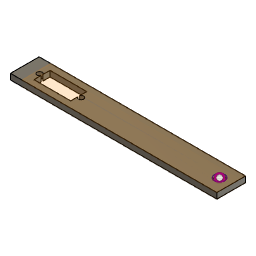
mechanical parts design (Autodesk Fusion 360 archive; units mm, degrees)
design "bar 1"
Autodesk Fusion 360 part; units mm, degrees
note: some values were not read from the file. Set by a fixed rule: which sketch regions a step uses.
sketch "Sketch1" plane through (0, 0, 0) normal (0, 1, 0) x (1, 0, 0)
  line L0 (0, 25) -> (170, 25)
  line L1 (170, 25) -> (170, 0)
  line L2 (170, 0) -> (0, 0)
  line L3 (0, 0) -> (0, 25)
  dimension "d1" = 170
  dimension "d2" = 25
  constraint horizontal L0
  constraint vertical L1
  constraint horizontal L2
  constraint vertical L3
  measures "d1" distance of L0.start L0.end
  measures "d2" distance of L0.end L1.end
extrude "Extrude1" add sketch "Sketch1" along normal blind 5
sketch "Sketch2" plane through (0, 5, 0) normal (0, 1, 0) x (-1, 0, 0)
  line L0 (0, 0) -> (-170, 0)
  line L1 (-170, 0) -> (-170, -25)
  line L2 (-170, -25) -> (0, -25)
  line L3 (0, -25) -> (0, 0)
  line L4 (0, -12.5) -> (-170, -12.5) construction
  line L5 (-5, -19.5) -> (-37, -19.5)
  line L6 (-37, -19.5) -> (-37, -5.5)
  line L7 (-37, -5.5) -> (-5, -5.5)
  line L8 (-5, -5.5) -> (-5, -19.5)
  line L9 (-13.6713, -25) -> (-13.6713, 0) construction
  dimension "d5" = 14
  dimension "d6" = 5.5
  dimension "d7" = 4
  dimension "d8" = 5
  dimension "d9" = 32
  dimension "d10" = 133
  constraint midpoint L3 L4.start
  constraint midpoint L1 L4.end
  constraint horizontal L5
  constraint vertical L6
  constraint horizontal L7
  constraint vertical L8
  constraint coincident L2 L9.start
  constraint coincident L0 L9.end
  constraint perpendicular L0 L9
  measures "d5" distance of L5.end L6.end
  measures "d6" distance of L2 L5
  measures "d8" distance of L3 L8
  measures "d9" distance of L5.start L5.end
  measures "d10" distance of L1 L6
extrude "Extrude2" cut sketch "Sketch2" against normal blind 5 contours L5 L6 L7 L8
sketch "Sketch3" plane through (0, 0, 0) normal (0, -1, 0) x (1, 0, 0)
  line L0 (37, -5.5) -> (37, -19.5)
  line L1 (37, -19.5) -> (5, -19.5)
  line L2 (5, -19.5) -> (5, -5.5)
  line L3 (5, -5.5) -> (37, -5.5)
  line L4 (170, 0) -> (0, 0)
  line L5 (0, 0) -> (0, -25)
  line L6 (0, -25) -> (170, -25)
  line L7 (170, -25) -> (170, 0)
sketch "Sketch4" plane through (0, 5, 0) normal (0, 1, 0) x (-1, 0, 0)
  line L0 (-37, -19.5) -> (-37, -5.5)
  line L1 (-37, -5.5) -> (-5, -5.5)
  line L2 (-5, -5.5) -> (-5, -19.5)
  line L3 (-5, -19.5) -> (-37, -19.5)
  line L4 (0, 0) -> (-170, 0)
  line L5 (-170, 0) -> (-170, -25)
  line L6 (-170, -25) -> (0, -25)
  line L7 (0, -25) -> (0, 0)
  circle A0 centre (-160, -12.3902) radius 4.5
  dimension "d13" = 170
  dimension "d14" = 25
  dimension "d15" = 16
  dimension "d16" = 32
  dimension "d17" = 9
  dimension "d18" = 10
  measures "d13" distance of L5 L7
  measures "d14" distance of L4.start L6.end
  measures "d16" distance of L0.start L2.end
  measures "d17" diameter of A0
  measures "d18" distance of L5 A0.centre
extrude "Extrude4" cut sketch "Sketch4" against normal blind 2 contours A0
sketch "Sketch5" plane through (0, 5, 0) normal (0, 1, 0) x (-1, 0, 0)
  line L0 (-37, -19.5) -> (-37, -5.5)
  line L1 (-37, -5.5) -> (-5, -5.5)
  line L2 (-5, -5.5) -> (-5, -19.5)
  line L3 (-5, -19.5) -> (-37, -19.5)
  line L4 (0, 0) -> (-170, 0)
  line L5 (-170, 0) -> (-170, -25)
  line L6 (-170, -25) -> (0, -25)
  line L7 (0, -25) -> (0, 0)
  circle A0 centre (-160, -12.3902) radius 4.5
sketch "Sketch6" plane through (0, 0, 0) normal (0, -1, 0) x (1, 0, 0)
sketch "Sketch7" plane through (0, 0, 0) normal (0, -1, 0) x (1, 0, 0)
sketch "Sketch8" plane through (0, 5, 0) normal (0, 1, 0) x (-1, 0, 0)
  circle A0 centre (-160, -12.3902) radius 2
  circle A1 centre (-160, -12.3902) radius 4.5
  dimension "d22" = 4
  constraint concentric A0 A1
  measures "d22" diameter of A0
extrude "Extrude5" cut sketch "Sketch8" against normal through all contours A0
sketch "Sketch9" plane through (0, 5, 0) normal (0, 1, 0) x (-1, 0, 0)
sketch "Sketch10" plane through (0, 5, 0) normal (0, 1, 0) x (-1, 0, 0)
  line L0 (-53, -12.5) -> (-21, -12.5) construction
  line L1 (-37, -19.5) -> (-37, -5.5) construction
  line L2 (-21, 7.5) -> (-21, -18.5) construction
  line L3 (-37, -5.5) -> (-5, -5.5) construction
  circle A0 centre (-39.1, -12.5) radius 2.25
  circle A1 centre (-2.9, -12.5) radius 2.25
  dimension "d24" = 4.5
  dimension "d25" = 18.1
  constraint horizontal L0
  constraint midpoint L0 L1
  constraint perpendicular L0 L2
  constraint midpoint L2 L3
  constraint coincident L0 A0.centre
  constraint symmetric L2 A0 A1
  measures "d24" diameter of A0
  measures "d25" distance of L2 A0.centre
extrude "Extrude6" cut sketch "Sketch10" against normal blind 5
sketch "Sketch11" plane through (0, 5, 0) normal (0, 1, 0) x (-1, 0, 0)
  line L0 (0, 0) -> (10, 0)
  line L1 (10, 0) -> (10, -25)
  line L2 (10, -25) -> (0, -25)
  line L3 (0, -25) -> (0, 0)
  dimension "d28" = 10
  dimension "d29" = 25
  constraint horizontal L0
  constraint vertical L1
  constraint horizontal L2
  constraint vertical L3
  constraint coincident L0.start L3.end
  measures "d28" distance of L0.start L0.end
  measures "d29" distance of L0.end L1.end
extrude "Extrude7" add sketch "Sketch11" against normal blind 5

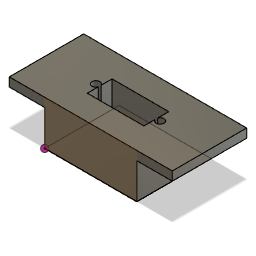
design "base"
Autodesk Fusion 360 part; units mm, degrees
sketch "Sketch1" plane through (0, 0, 0) normal (0, 1, 0) x (1, 0, 0)
  line L0 (0, 0) -> (52, 0)
  line L1 (52, 0) -> (52, 42)
  line L2 (52, 42) -> (0, 42)
  line L3 (0, 42) -> (0, 0)
  dimension "d1" = 42
  dimension "d2" = 52
  constraint horizontal L0
  constraint vertical L1
  constraint horizontal L2
  constraint vertical L3
  constraint coincident L0.start L3.end
  measures "d1" distance of L0.start L2.end
  measures "d2" distance of L1.end L2.end
extrude "Extrude2" add sketch "Sketch1" along normal blind 25
sketch "Sketch2" plane through (0, 0, 0) normal (0, 0, 1) x (1, 0, 0)
  line L0 (0, 0) -> (52, 0)
  line L1 (52, 0) -> (52, 25)
  line L2 (52, 25) -> (0, 25)
  line L3 (0, 25) -> (0, 0)
sketch "Sketch3" plane through (0, 25, 0) normal (0, 1, 0) x (-1, 0, 0)
  line L0 (0, -42) -> (0, 0)
  line L1 (0, 0) -> (-52, 0)
  line L2 (-52, 0) -> (-52, -42)
  line L3 (-52, -42) -> (0, -42)
  line L4 (-10, -28) -> (-42, -28)
  line L5 (-42, -28) -> (-42, -14)
  line L6 (-42, -14) -> (-10, -14)
  line L7 (-10, -14) -> (-10, -28)
  line L8 (0, -21) -> (-52, -21) construction
  line L9 (-10, -21) -> (-42, -21) construction
  line L10 (-26, -42) -> (-26, 0) construction
  dimension "d7" = 32
  dimension "d8" = 14
  constraint horizontal L4
  constraint vertical L5
  constraint horizontal L6
  constraint vertical L7
  constraint midpoint L0 L8.start
  constraint midpoint L2 L8.end
  constraint midpoint L7 L9.start
  constraint midpoint L5 L9.end
  constraint midpoint L3 L10.start
  constraint midpoint L1 L10.end
  constraint midpoint L9 L10
  measures "d7" distance of L4.start L4.end
  measures "d8" distance of L4.end L5.end
extrude "Extrude3" cut sketch "Sketch3" against normal blind 25 contours L4 L5 L6 L7
sketch "Sketch6" plane through (0, 25, 0) normal (0, 1, 0) x (-1, 0, 0)
  line L0 (-42, -28) -> (-42, -14)
  line L1 (-42, -14) -> (-10, -14)
  line L2 (-10, -14) -> (-10, -28)
  line L3 (-10, -28) -> (-42, -28)
  line L4 (0, -42) -> (0, 0)
  line L5 (0, 0) -> (-52, 0)
  line L6 (-52, 0) -> (-52, -42)
  line L7 (-52, -42) -> (0, -42)
  circle A0 centre (-7.9, -21) radius 2.25
  line L8 (-26, -42) -> (-26, 0) construction
  circle A1 centre (-44.1, -21) radius 2.25
  dimension "d11" = 18.1
  dimension "d12" = 4.5
  constraint midpoint L7 L8.start
  constraint midpoint L5 L8.end
  constraint symmetric A0 L8 A1
  measures "d11" distance of A0.centre L8
  measures "d12" diameter of A0
extrude "Extrude4" cut sketch "Sketch6" against normal blind 25 contours L0 A1 | L2 A0 picked at (-45.0271, -20.3199) picked at (-8.55, -21)
sketch "Sketch7" plane through (0, 25, 0) normal (0, 1, 0) x (-1, 0, 0)
  line L0 (0, -42) -> (0, 0)
  line L1 (0, 0) -> (-52, 0)
  line L2 (-52, 0) -> (-52, -42)
  line L3 (-52, -42) -> (0, -42)
  arc A0 (-10, -21.8078) -> (-10, -20.1922) centre (-7.9, -21) ccw
  line L4 (-10, -21.8078) -> (-10, -28)
  line L5 (-10, -28) -> (-42, -28)
  line L6 (-42, -28) -> (-42, -21.8078)
  arc A1 (-42, -20.1922) -> (-42, -21.8078) centre (-44.1, -21) ccw
  line L7 (-42, -20.1922) -> (-42, -14)
  line L8 (-42, -14) -> (-10, -14)
  line L9 (-10, -14) -> (-10, -20.1922)
  line L10 (-52, -42) -> (-72, -42)
  line L11 (-72, -42) -> (-72, 0)
  line L12 (-72, 0) -> (-52, 0)
  line L13 (-52, 0) -> (-52, -42)
  line L14 (-26, -42) -> (-26, 0) construction
  line L15 (0, -42) -> (20, -42)
  line L16 (20, -42) -> (20, 0)
  line L17 (20, 0) -> (0, 0)
  line L18 (0, 0) -> (0, -42)
  dimension "d15" = 20
  constraint horizontal L10
  constraint vertical L11
  constraint horizontal L12
  constraint vertical L13
  constraint coincident L2.end L3.start
  constraint midpoint L3 L14.start
  constraint midpoint L1 L14.end
  constraint symmetric L2.end L14 L0.start
  constraint symmetric L10.end L14 L15.end
  constraint symmetric L11.end L14 L16.end
  constraint symmetric L1.end L14 L0.end
  measures "d15" distance of L2.end L10.end
extrude "Extrude5" add sketch "Sketch7" against normal blind 5 contours L0 L15 L16 L17 L18 | L2 L10 L11 L12 L13

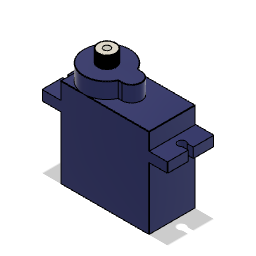
design "Servo Motor SG90"
Autodesk Fusion 360 part; units mm, degrees
sketch "Sketch1" plane through (0, 0, 0) normal (0, 0, 1) x (1, 0, 0)
  line L0 (0, 0) -> (0, 4.3)
  line L1 (0, -18.4) -> (0, -2.5)
  line L2 (0, -2.5) -> (-4.7, -2.5)
  line L3 (-4.7, -2.5) -> (-4.7, 0)
  line L4 (-4.7, 0) -> (0, 0)
  line L5 (22.5, 0) -> (22.5, 4.3)
  line L6 (27.2, 0) -> (22.5, 0)
  line L7 (27.2, -2.5) -> (27.2, 0)
  line L8 (22.5, -2.5) -> (27.2, -2.5)
  line L9 (22.5, -18.4) -> (22.5, -2.5)
  line L10 (0, -18.4) -> (22.5, -18.4)
  line L11 (0, 4.3) -> (22.5, 4.3)
  dimension "d2" = 4.7
  dimension "d3" = 2.5
  dimension "d4" = 15.9
  dimension "d5" = 22.7
  dimension "d7" = 22.5
  dimension "d9" = 22.5
  dimension "d10" = 15.9
  constraint coincident L0.start L4.end
  constraint vertical L0
  constraint perpendicular L1 L2
  constraint perpendicular L2 L3
  constraint perpendicular L0 L4
  constraint perpendicular L9 L10
  constraint perpendicular L5 L11
  constraint parallel L1 L9
  constraint parallel L0 L5
  constraint parallel L6 L8
  constraint parallel L2 L4
  measures "d2" distance of L3.end L0.start
  measures "d3" distance of L2.end L3.end
  measures "d4" distance of L1.start L1.end
  measures "d5" distance of L0.end L1.start
  measures "d7" distance of L0.end L5.end
  measures "d9" distance of L1.start L9.start
  measures "d10" distance of L8.start L9.start
extrude "Extrude1" add sketch "Sketch1" along normal blind 11.8 contours L0 L1 L2 L3 L4 L5 L6 L7 L8 L9 L10 L11 picked at (7.5, -7.8) makes body 1
sketch "Sketch6" plane through (0, 4.3, 0) normal (0, 1, 0) x (-1, 0, 0)
  line L0 (-22.5, 0) -> (0, 0)
  line L1 (0, 0) -> (0, 11.8)
  line L2 (0, 11.8) -> (-22.5, 11.8)
  line L3 (-22.5, 11.8) -> (-22.5, 0)
  line L4 (-11.244156, 3.4) -> (-12.2, 3.4)
  arc A0 (-12.2, 8.4) -> (-12.2, 3.4) centre (-12.2, 5.9) ccw
  line L5 (-12.2, 8.4) -> (-11.244156, 8.4)
  arc A1 (-11.244156, 3.4) -> (-11.244156, 8.4) centre (-5.9, 5.9) ccw
  dimension "d69" = 11.8
  dimension "d71" = 5
  dimension "d72" = 3.4
  dimension "d73" = 10.3
  constraint tangent L0 A1
  constraint tangent L1 A1
  constraint parallel L2 L4
  constraint tangent L4 A0
  constraint tangent A0 L5
  constraint parallel L4 L5
  measures "d69" diameter of A1
  measures "d71" distance of L4 L5
  measures "d72" distance of L0 L4
  measures "d73" distance of L3 A0.centre
extrude "Extrude9" add sketch "Sketch6" along normal blind 4 contours L4 A0 L5 A1 picked at (-7.380628, 5.376962) bodies 1
sketch "Sketch7" plane through (0, 8.3, 0) normal (0, 1, 0) x (-1, 0, 0)
  arc A0 (-12.2, 8.4) -> (-12.2, 3.4) centre (-12.2, 5.9) ccw
  line L0 (-12.2, 3.4) -> (-11.244156, 3.4)
  arc A1 (-11.244156, 3.4) -> (-11.244156, 8.4) centre (-5.9, 5.9) ccw
  line L1 (-11.244156, 8.4) -> (-12.2, 8.4)
  circle A2 centre (-5.9, 5.9) radius 2.3
  line L2 (-5.9, 11.8) -> (0, 11.8)
  dimension "d77" = 4.6
  constraint concentric A1 A2
  measures "d77" diameter of A2
extrude "Extrude10" add sketch "Sketch7" along normal blind 3.2 separate body contours A2 picked at (-7.201969, 6.065119) makes body 2
sketch "Sketch8" plane through (0, 11.5, 0) normal (0, 1, 0) x (-1, 0, 0)
  circle A0 centre (-5.9, 5.9) radius 2.3
  circle A1 centre (-5.9, 5.9) radius 0.85
  line L0 (-5.927716, 8.066913) -> (-6, 8.241421)
  line L1 (-6, 8.241421) -> (-5.8, 8.241421)
  line L2 (-5.8, 8.241421) -> (-5.872284, 8.066913)
  arc A2 (-5.927716, 8.066913) -> (-5.872284, 8.066913) centre (-5.9, 8.078394) ccw
  point P0 (-5.9, 8)
  dimension "d81" = 1.7
  dimension "d84" = 0.1
  dimension "d85" = 0.1
  dimension "d86" = 45
  dimension "d88" = 2.1
  dimension "d94" = 0.03
  constraint concentric A0 A1
  constraint coincident P0 L0
  constraint coincident P0 L2
  constraint tangent L0 A2
  constraint tangent L2 A2
  measures "d81" diameter of A1
  measures "d86" angle of L0 L2
  measures "d88" distance of A0.centre P0
  measures "d94" radius of A2
extrude "Extrude11" cut sketch "Sketch8" against normal blind 3.2 contours A1 picked at (-6.010624, 5.693552) bodies 2
extrude "Extrude12" cut sketch "Sketch8" against normal blind 3.2 contours A0 L0 L2 A2 | A0 L0 L1 L2 picked at (-5.909139, 8.111221) picked at (-5.909139, 8.22756) bodies 2
fillet "Fillet4" radius 0.01 2 edges at (5.817766, 9.9, 8.198529) (5.982234, 9.9, 8.198529) on bodies 2
pattern_circular "C-Pattern2" count 80 over 360 about axis through (5.9, 11.5, 5.9) along (0, 1, 0) of "Extrude12", "Fillet4"
sketch "Sketch9" plane through (0, 0, 0) normal (0, 1, 0) x (-1, 0, 0)
  line L0 (0, 0) -> (4.7, 0)
  line L1 (4.7, 0) -> (4.7, 11.8)
  line L2 (4.7, 11.8) -> (0, 11.8)
  line L3 (0, 11.8) -> (0, 0)
  line L4 (3, 5.25) -> (4.7, 5.25)
  line L5 (3, 6.55) -> (4.7, 6.55)
  arc A0 (3.159934, 6.55) -> (3.159934, 5.25) centre (2.4, 5.9) ccw
  line L6 (-27.2, 0) -> (-27.2, 11.8)
  line L7 (-27.2, 11.8) -> (-22.5, 11.8)
  line L8 (-27.2, 6.55) -> (-25.5, 6.55)
  line L9 (-27.2, 5.25) -> (-25.5, 5.25)
  arc A1 (-25.659934, 5.25) -> (-25.659934, 6.55) centre (-24.9, 5.9) ccw
  dimension "d95" = 2
  dimension "d96" = 2.3
  dimension "d97" = 1.3
  dimension "d99" = 5.9
  dimension "d100" = 0.65
  dimension "d101" = 2
  dimension "d102" = 2.3
  dimension "d103" = 5.9
  dimension "d104" = 1.3
  dimension "d105" = 0.65
  constraint coincident L1 L4.end
  constraint perpendicular L1 L4
  constraint coincident L1 L5.end
  constraint perpendicular L1 L5
  constraint coincident L6 L8.start
  constraint perpendicular L6 L8
  constraint coincident L6 L9.start
  constraint perpendicular L6 L9
  measures "d95" diameter of A0
  measures "d96" distance of L1 A0.centre
  measures "d97" distance of L4 L5
  measures "d99" distance of L2 A0.centre
  measures "d100" distance of A0.centre L5
  measures "d101" diameter of A1
  measures "d102" distance of A1.centre L6
  measures "d103" distance of A1.centre L7
  measures "d104" distance of L8 L9
  measures "d105" distance of A1.centre L8
extrude "Extrude13" cut sketch "Sketch9" against normal through all contours L1 L4 L5 A0 | L6 L8 L9 A1 picked at (3.673289, 6.116667) picked at (-25.074196, 5.924564) bodies 1
fillet "Fillet5" radius 0.1 27 edges at (0, 8.3, 5.9) (11.722078, 8.3, 8.4) (14.7, 8.3, 5.9) (11.722078, 8.3, 3.4) (14.2, 4.3, 11.8) (22.5, 4.3, 5.9) (14.2, 4.3, 0) (2.95, 4.3, 11.8) (0, 4.3, 8.85) (0, 4.3, 2.95) (2.95, 4.3, 0) (-4.7, -1.25, 11.8) (11.25, -18.4, 11.8) (0, -18.4, 5.9) (11.25, -18.4, 0) (22.5, -18.4, 5.9) (22.5, -10.45, 0) (22.5, -10.45, 11.8) (27.2, -1.25, 11.8) (27.2, -1.25, 0) (22.5, 2.15, 11.8) (22.5, 2.15, 0) (0, -10.45, 0) (-4.7, -1.25, 0) (0, 2.15, 0) (0, 2.15, 11.8) (0, -10.45, 11.8) on bodies 1
equation "d85 = d84"

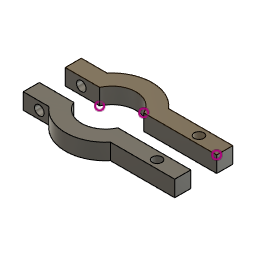
design "end joiint pen holder"
Autodesk Fusion 360 part; units mm, degrees
sketch "Sketch1" plane through (0, 0, 0) normal (0, 1, 0) x (1, 0, 0)
  line L0 (6.8573, 3.0376) -> (29.5732, 3.0376)
  line L1 (29.5732, 3.0376) -> (29.5732, 8.0376)
  line L2 (29.5732, 8.0376) -> (9.5732, 8.0376)
  line L3 (0, -7.5) -> (0, 7.5) construction
  line L4 (-29.5732, 8.0376) -> (-9.5732, 8.0376)
  line L5 (-6.8573, 3.0376) -> (-29.5732, 3.0376)
  line L6 (-29.5732, 3.0376) -> (-29.5732, 8.0376)
  arc A0 (9.5732, 8.0376) -> (-9.5732, 8.0376) centre (0, 0) ccw
  arc A1 (6.8573, 3.0376) -> (-6.8573, 3.0376) centre (0, 0) ccw
  dimension "d1" = 15
  dimension "d2" = 25
  dimension "d3" = 20
  dimension "d4" = 5
  dimension "d24" = 3.0376
  constraint coincident A0.centre A1.centre
  constraint concentric A0 A1
  constraint horizontal L0
  constraint vertical L1
  constraint horizontal L2
  constraint coincident L3.end A1
  constraint vertical L3
  constraint midpoint A0.centre L3
  constraint symmetric L0.start L3 L5.start
  constraint symmetric L0.end L3 L5.end
  constraint symmetric L1.end L3 L4.start
  constraint symmetric L2.end L3 L4.end
  measures "d1" diameter of A1
  measures "d2" diameter of A0
  measures "d3" distance of L1.end L2.end
  measures "d4" distance of L0.end L1.end
  measures "d24" distance of A0.centre L0
sketch "Sketch2" plane through (0, 0, 0) normal (0, 1, 0) x (1, 0, 0)
sketch "Sketch3" plane through (0, 0, 0) normal (0, 1, 0) x (1, 0, 0)
  point P0 (-6.8573, 3.0376)
extrude "Extrude1" add sketch "Sketch1" along normal blind 5 makes body 1
sketch "Sketch4" plane through (0, 5, 0) normal (0, 1, 0) x (-1, 0, 0)
  line L0 (-29.5732, -3.0376) -> (-29.5732, -8.0376)
  line L1 (-29.5732, -8.0376) -> (-9.5732, -8.0376)
  arc A0 (-9.5732, -8.0376) -> (9.5732, -8.0376) centre (0, 0) ccw
  line L2 (9.5732, -8.0376) -> (29.5732, -8.0376)
  line L3 (29.5732, -8.0376) -> (29.5732, -3.0376)
  line L4 (29.5732, -3.0376) -> (6.8573, -3.0376)
  arc A1 (-6.8573, -3.0376) -> (6.8573, -3.0376) centre (0, 0) ccw
  line L5 (-6.8573, -3.0376) -> (-29.5732, -3.0376)
  line L6 (29.5732, -8.0376) -> (17.5732, -8.0376)
  line L7 (17.5732, -8.0376) -> (17.5732, -3.0376)
  line L8 (17.5732, -3.0376) -> (29.5732, -3.0376)
  line L9 (29.5732, -3.0376) -> (29.5732, -8.0376)
  dimension "d8" = 12
  constraint horizontal L6
  constraint vertical L7
  constraint horizontal L8
  constraint vertical L9
  constraint coincident L4 L7.end
  constraint coincident L2.end L3.start
  measures "d8" distance of L2.end L6.end
extrude "Extrude2" cut sketch "Sketch4" against normal blind 5 contours L2 L3 L4 L6 L7 L8 L9 bodies 1
sketch "Sketch5" plane through (0, 5, 0) normal (0, 1, 0) x (-1, 0, 0)
  line L0 (17.5732, -8.0376) -> (17.5732, -3.0376)
  line L1 (17.5732, -3.0376) -> (6.8573, -3.0376)
  arc A0 (-6.8573, -3.0376) -> (6.8573, -3.0376) centre (0, 0) ccw
  line L2 (-6.8573, -3.0376) -> (-29.5732, -3.0376)
  line L3 (-29.5732, -3.0376) -> (-29.5732, -8.0376)
  line L4 (-29.5732, -8.0376) -> (-9.5732, -8.0376)
  arc A1 (-9.5732, -8.0376) -> (9.5732, -8.0376) centre (0, 0) ccw
  line L5 (9.5732, -8.0376) -> (17.5732, -8.0376)
  dimension "d11" = 2.5
sketch "Sketch6" plane through (0, 0, -3.0376) normal (0, 0, 1) x (1, 0, 0)
  line L0 (-17.5732, 5) -> (-17.5732, 0)
  line L1 (-17.5732, 0) -> (-6.8573, 0)
  line L2 (-6.8573, 0) -> (-6.8573, 5)
  line L3 (-6.8573, 5) -> (-17.5732, 5)
  circle A0 centre (-12.5732, 2.5) radius 1.5
  dimension "d12" = 2.5
  dimension "d13" = 3
  dimension "d14" = 5
  measures "d12" distance of L3 A0.centre
  measures "d13" diameter of A0
  measures "d14" distance of L0 A0.centre
extrude "Extrude3" cut sketch "Sketch6" against normal blind 5 contours A0 bodies 1
sketch "Sketch7" plane through (0, 5, 0) normal (0, 1, 0) x (-1, 0, 0)
  circle A0 centre (-21.5732, -5.5046) radius 1.5
  line L0 (-29.5732, -3.0376) -> (-29.5732, -8.0376)
  dimension "d17" = 3
  dimension "d18" = 8
  measures "d17" diameter of A0
  measures "d18" distance of A0.centre L0
extrude "Extrude4" cut sketch "Sketch7" against normal blind 5 bodies 1
sketch "Sketch8" plane through (0, 5, 0) normal (0, 1, 0) x (-1, 0, 0)
  point P0 (-29.5732, -3.0376)
  point P1 (-6.8573, -3.0376)
  dimension "d21" = 22.7159
  measures "d21" distance of P0 P1
mirror "Mirror1" about plane through (0, 0, 0) normal (0, 0, 1) of bodies 1 makes body 2
move_body "Move1" bodies 2 to x (1, 0, 0) y (0, 1, 0) z (0, 0, 1) at (0, 0, 4)
move_body "Move2" bodies 2 to x (1, 0, 0) y (0, 1, 0) z (0, 0, 1) at (0, 0, -2)

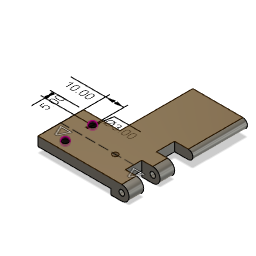
design "bar 3"
Autodesk Fusion 360 part; units mm, degrees
sketch "Sketch1" plane through (0, 0, 0) normal (0, 1, 0) x (1, 0, 0)
  line L0 (0, 0) -> (40, 0)
  line L1 (40, 0) -> (40, 25)
  line L2 (40, 25) -> (0, 25)
  line L3 (0, 25) -> (0, 0)
  dimension "d1" = 25
  dimension "d2" = 40
  constraint horizontal L0
  constraint vertical L1
  constraint horizontal L2
  constraint vertical L3
  constraint coincident L0.start L3.end
  measures "d1" distance of L0.start L2.end
  measures "d2" distance of L0.start L0.end
  measures "d38" diameter of L0.start
extrude "Extrude1" add sketch "Sketch1" along normal blind 5
sketch "Sketch2" plane through (0, 5, 0) normal (0, 1, 0) x (-1, 0, 0)
  line L0 (0, -25) -> (0, 0)
  line L1 (0, 0) -> (-40, 0)
  line L2 (-40, 0) -> (-40, -25)
  line L3 (-40, -25) -> (0, -25)
  line L4 (-40, -25) -> (-50, -25)
  line L5 (-50, -25) -> (-50, 0)
  line L6 (-50, 0) -> (-40, 0)
  line L7 (-40, 0) -> (-40, -25)
  dimension "d5" = 10
  dimension "d6" = 25
  constraint horizontal L4
  constraint vertical L5
  constraint horizontal L6
  constraint vertical L7
  constraint coincident L2.end L3.start
  measures "d5" distance of L2.end L4.end
  measures "d6" distance of L4.end L5.end
extrude "Extrude2" add sketch "Sketch2" against normal blind 8 contours L2 L4 L5 L6 L7
fillet "Fillet2" radius 4 2 edges at (50, 5, -12.5) (50, -3, -12.5)
sketch "Sketch4" plane through (0, 0, 0) normal (0, 0, 1) x (1, 0, 0)
  arc A0 (46, -3) -> (46, 5) centre (46, 1) ccw
  line L0 (46, 5) -> (0, 5)
  line L1 (0, 5) -> (0, 0)
  line L2 (0, 0) -> (40, 0)
  line L3 (40, 0) -> (40, -3)
  line L4 (40, -3) -> (46, -3)
  circle A1 centre (46, 1) radius 1.5
  dimension "d14" = 3
  constraint concentric A0 A1
  measures "d14" diameter of A1
extrude "Extrude3" cut sketch "Sketch4" against normal blind 25 contours A1
sketch "Sketch5" plane through (0, -3, 0) normal (0, -1, 0) x (1, 0, 0)
  line L0 (46, -25) -> (46, 0)
  line L1 (46, 0) -> (40, 0)
  line L2 (40, 0) -> (40, -25)
  line L3 (40, -25) -> (46, -25)
  line L4 (40, -8) -> (50, -8)
  line L5 (50, -8) -> (50, -17)
  line L6 (50, -17) -> (40, -17)
  line L7 (40, -17) -> (40, -8)
  dimension "d17" = 9
  constraint horizontal L4
  constraint vertical L5
  constraint horizontal L6
  constraint vertical L7
  constraint coincident L2 L4.start
  constraint midpoint L2 L7
  measures "d17" distance of L4.end L5.end
extrude "Extrude4" cut sketch "Sketch5" against normal blind 8 contours L0 L2 L4 L6 L7 | L0 L4 L5 L6
sketch "Sketch6" plane through (0, 0, 0) normal (0, -1, 0) x (1, 0, 0)
  line L0 (0, 0) -> (0, -25)
  line L1 (0, -25) -> (40, -25)
  line L2 (40, -25) -> (40, -17)
  line L3 (40, -17) -> (40, -8)
  line L4 (40, -8) -> (40, 0)
  line L5 (40, 0) -> (0, 0)
  circle A0 centre (30, -12.5) radius 1.5
  dimension "d20" = 12.5
  dimension "d21" = 3
  dimension "d24" = 10
  measures "d20" distance of L5 A0.centre
  measures "d21" diameter of A0
  measures "d24" distance of L3 A0.centre
extrude "Extrude5" cut sketch "Sketch6" against normal blind 5 contours A0
sketch "Sketch8" plane through (0, 5, 0) normal (0, 1, 0) x (-1, 0, 0)
  circle A0 centre (-30, -12.5) radius 1.5
  line L0 (-40, -17) -> (-46, -17)
  line L1 (-46, -17) -> (-46, -25)
  line L2 (-46, -25) -> (0, -25)
  line L3 (0, -25) -> (0, 0)
  line L4 (0, 0) -> (-46, 0)
  line L5 (-46, 0) -> (-46, -8)
  line L6 (-46, -8) -> (-40, -8)
  line L7 (-40, -8) -> (-40, -17)
  line L8 (-20, -25) -> (-40, -25)
  line L9 (-40, -25) -> (-40, -30)
  line L10 (-20, -30) -> (-20, -25)
  line L11 (-50, -30) -> (-50, -65)
  line L12 (-50, -65) -> (-20, -65)
  line L13 (-20, -65) -> (-20, -30)
  line L14 (-40, -30) -> (-50, -30)
  dimension "d27" = 5
  dimension "d28" = 30
  dimension "d29" = 20
  dimension "d30" = 35
  constraint horizontal L8
  constraint vertical L9
  constraint vertical L10
  constraint coincident L2 L8.start
  constraint vertical L11
  constraint horizontal L12
  constraint vertical L13
  constraint perpendicular L11 L14
  measures "d27" distance of L8.end L9.end
  measures "d28" distance of L10.start L11.start
  measures "d29" distance of L9.end L10.start
  measures "d30" distance of L11.start L11.end
extrude "Extrude6" add sketch "Sketch8" against normal blind 5 contours L2 L8 L9 L10 L11 L12 L13 L14
fillet "Fillet3" radius 2.5 2 edges at (50, 0, -47.5) (50, 5, -47.5)
sketch "Sketch9" plane through (0, 5, 0) normal (0, 1, 0) x (-1, 0, 0)
  line L0 (-47.5, -30) -> (-47.5, -65)
  line L1 (-47.5, -65) -> (-20, -65)
  line L2 (-20, -65) -> (-20, -25)
  line L3 (-20, -25) -> (0, -25)
  line L4 (0, -25) -> (0, 0)
  line L5 (0, 0) -> (-46, 0)
  line L6 (-46, 0) -> (-46, -8)
  line L7 (-46, -8) -> (-40, -8)
  line L8 (-40, -8) -> (-40, -17)
  line L9 (-40, -17) -> (-46, -17)
  line L10 (-46, -17) -> (-46, -25)
  line L11 (-46, -25) -> (-40, -25)
  line L12 (-40, -25) -> (-40, -30)
  line L13 (-40, -30) -> (-47.5, -30)
  circle A0 centre (-30, -12.5) radius 1.5
  line L14 (-40, -30) -> (-50, -30)
  line L15 (-50, -30) -> (-50, -35)
  line L16 (-50, -35) -> (-40, -35)
  line L17 (-40, -35) -> (-40, -30)
  dimension "d34" = 5
  dimension "d35" = 10
  constraint horizontal L14
  constraint vertical L15
  constraint horizontal L16
  constraint vertical L17
  constraint coincident L12.end L13.start
  measures "d34" distance of L12.end L16.end
  measures "d35" distance of L15.end L16.end
extrude "Extrude7" cut sketch "Sketch9" against normal blind 5 contours L0 L13 L14 L16 L17 | L0 L14 L15 L16
sketch "Sketch10" plane through (0, 5, 0) normal (0, 1, 0) x (-1, 0, 0)
  line L0 (-40, -35) -> (-47.5, -35)
  line L1 (-47.5, -35) -> (-47.5, -65)
  line L2 (-47.5, -65) -> (-20, -65)
  line L3 (-20, -65) -> (-20, -25)
  line L4 (-20, -25) -> (0, -25)
  line L5 (0, -25) -> (0, 0)
  line L6 (0, 0) -> (-46, 0)
  line L7 (-46, 0) -> (-46, -8)
  line L8 (-46, -8) -> (-40, -8)
  line L9 (-40, -8) -> (-40, -17)
  line L10 (-40, -17) -> (-46, -17)
  line L11 (-46, -17) -> (-46, -25)
  line L12 (-46, -25) -> (-40, -25)
  line L13 (-40, -25) -> (-40, -35)
  circle A0 centre (-30, -12.5) radius 1.5
  circle A1 centre (-10, -20) radius 1.5
  line L14 (-40, -12.5) -> (0, -12.5) construction
  circle A2 centre (-10, -5) radius 1.5
  dimension "d38" = 3
  dimension "d39" = 10
  dimension "d42" = 5
  constraint midpoint L9 L14.start
  constraint midpoint L5 L14.end
  constraint symmetric A1 L14 A2
  measures "d38" diameter of A1
  measures "d39" distance of L5 A1.centre
  measures "d42" distance of L4 A1.centre
extrude "Extrude9" cut sketch "Sketch10" against normal blind 5 contours A1 | A2
extrude "Extrude8" cut sketch "Sketch10" against normal blind 5 contours A1
sketch "Sketch11" plane through (0, 5, 0) normal (0, 1, 0) x (-1, 0, 0)
  line L0 (-40, -35) -> (-47.5, -35)
  line L1 (-47.5, -35) -> (-47.5, -65)
  line L2 (-47.5, -65) -> (-20, -65)
  line L3 (-20, -65) -> (-20, -25)
  line L4 (-20, -25) -> (0, -25)
  line L5 (0, -25) -> (0, 0)
  line L6 (0, 0) -> (-46, 0)
  line L7 (-46, 0) -> (-46, -8)
  line L8 (-46, -8) -> (-40, -8)
  line L9 (-40, -8) -> (-40, -17)
  line L10 (-40, -17) -> (-46, -17)
  line L11 (-46, -17) -> (-46, -25)
  line L12 (-46, -25) -> (-40, -25)
  line L13 (-40, -25) -> (-40, -35)
  circle A0 centre (-30, -12.5) radius 1.5
  circle A1 centre (-10, -20) radius 1.5
  circle A2 centre (-10, -5) radius 1.5
